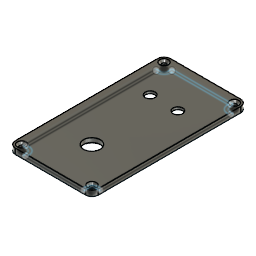
assembly (Autodesk Fusion 360 archive; units mm, degrees)
design "Couvercle"
part number: 2025-12-11-08-38-01-153
Autodesk Fusion 360 part; units mm, degrees
sketch "Esquisse1" plane through (0, 0, 0) normal (0, 0, 1) x (1, 0, 0)
  line L0 (0, 0) -> (60, 0)
  line L1 (60, 0) -> (60, -112)
  line L2 (60, -112) -> (0, -112)
  line L3 (0, -112) -> (0, 0)
  dimension "d1" = 60
  dimension "d2" = 112
  constraint horizontal L0
  constraint vertical L1
  constraint horizontal L2
  constraint vertical L3
  constraint coincident L0.start L3.end
  measures "d1" distance of L0.start L0.end
  measures "d2" distance of L0.start L2.end
extrude "Extrusion1" add sketch "Esquisse1" along normal blind 4
sketch "Esquisse2" plane through (0, 0, 4) normal (0, 0, 1) x (-1, 0, 0)
  line L0 (0, 112) -> (-60, 112)
  line L1 (-60, 112) -> (-60, 0)
  line L2 (-60, 0) -> (0, 0)
  line L3 (0, 0) -> (0, 112)
  circle A0 centre (-4.6, 4.6) radius 1.6
  circle A1 centre (-4.6, 4.6) radius 1.6
  circle A2 centre (-55.4, 4.6) radius 1.6
  circle A3 centre (-4.6, 107.4) radius 1.6
  circle A4 centre (-55.4, 107.4) radius 1.6
  dimension "d5" = 3.2
  dimension "d6" = 4.6
  dimension "d7" = 4.6
  dimension "d8" = 3.2
  dimension "d9" = 3.2
  dimension "d10" = 4.6
  dimension "d11" = 4.6
  dimension "d12" = 3.2
  dimension "d13" = 4.6
  dimension "d14" = 4.6
  dimension "d15" = 3.2
  dimension "d16" = 4.6
  dimension "d17" = 4.6
  measures "d5" diameter of A0
  measures "d6" distance of L3 A0.centre
  measures "d7" distance of L2 A0.centre
  measures "d8" diameter of A1
  measures "d9" diameter of A2
  measures "d10" distance of L1 A2.centre
  measures "d11" distance of L2 A2.centre
  measures "d12" diameter of A3
  measures "d13" distance of L0 A3.centre
  measures "d14" distance of L3 A3.centre
  measures "d15" diameter of A4
  measures "d16" distance of L1 A4.centre
  measures "d17" distance of L0 A4.centre
hole "Perçage1" at (4.6, -4.6, 4) at (55.4, -4.6, 4) at (55.4, -107.4, 4) at (4.6, -107.4, 4) direction (0, 0, -1) diameter 3.2 depth 25 tip angle 118 countersink diameter 6.3 countersink angle 90
fillet "Congé1" radius 4.6 4 edges at (0, 0, 2) (60, 0, 2) (60, -112, 2) (0, -112, 2)
sketch "Esquisse3" plane through (0, 0, 0) normal (0, 0, -1) x (1, 0, 0)
  circle A0 centre (55.4, 107.4) radius 1.6
  circle A1 centre (4.6, 4.6) radius 1.6
  circle A2 centre (55.4, 4.6) radius 1.6
  circle A3 centre (4.6, 107.4) radius 1.6
  arc A4 (4.6, 112) -> (0, 107.4) centre (4.6, 107.4) ccw
  line L0 (0, 107.4) -> (0, 4.6)
  arc A5 (0, 4.6) -> (4.6, 0) centre (4.6, 4.6) ccw
  line L1 (4.6, 0) -> (55.4, 0)
  arc A6 (55.4, 0) -> (60, 4.6) centre (55.4, 4.6) ccw
  line L2 (60, 4.6) -> (60, 107.4)
  arc A7 (60, 107.4) -> (55.4, 112) centre (55.4, 107.4) ccw
  line L3 (55.4, 112) -> (4.6, 112)
  line L4 (8.9, 110) -> (51.6, 110)
  line L5 (2, 8.7) -> (2, 103.1)
  line L6 (52.1, 107.4) -> (52.1, 109.5)
  arc A8 (52.1, 107.4) -> (55.4467, 104.1003) centre (55.4, 107.4) ccw
  line L7 (55.3533, 104.1003) -> (57.5, 104.1003)
  arc A9 (52.1, 109.5) -> (51.6, 110) centre (51.6, 109.5) ccw
  arc A10 (58, 103.6003) -> (57.5, 104.1003) centre (57.5, 103.6003) ccw
  line L8 (7.9, 109) -> (7.9, 107.4)
  line L9 (3, 104.1) -> (4.6, 104.1)
  arc A11 (4.6, 104.1) -> (7.9, 107.4) centre (4.6, 107.4) ccw
  line L10 (3, 7.7) -> (4.6, 7.7)
  line L11 (7.7, 3) -> (7.7, 4.6)
  arc A12 (7.7, 4.6) -> (4.6, 7.7) centre (4.6, 4.6) ccw
  line L12 (57, 7.7) -> (55.4, 7.7)
  line L13 (52.3, 3) -> (52.3, 4.6)
  arc A13 (55.4, 7.7) -> (52.3, 4.6) centre (55.4, 4.6) ccw
  line L14 (58, 103.6003) -> (58, 8.7)
  line L15 (51.3, 2) -> (8.7, 2)
  arc A14 (8.9, 110) -> (7.9, 109) centre (8.9, 109) ccw
  arc A15 (3, 104.1) -> (2, 103.1) centre (3, 103.1) ccw
  arc A16 (2, 8.7) -> (3, 7.7) centre (3, 8.7) ccw
  arc A17 (7.7, 3) -> (8.7, 2) centre (8.7, 3) ccw
  arc A18 (51.3, 2) -> (52.3, 3) centre (51.3, 3) ccw
  arc A19 (57, 7.7) -> (58, 8.7) centre (57, 8.7) ccw
  line L16 (55.4592, 102.1003) -> (56, 102.1003)
  line L17 (56, 102.1003) -> (56, 9.7)
  line L18 (56, 9.7) -> (55.4, 9.7)
  arc A20 (55.4, 9.7) -> (50.3, 4.6) centre (55.4, 4.6) ccw
  line L19 (50.3, 4) -> (50.3, 4.6)
  line L20 (50.3, 4) -> (9.7, 4)
  line L21 (9.7, 4) -> (9.7, 4.6)
  arc A21 (9.7, 4.6) -> (4.6, 9.7) centre (4.6, 4.6) ccw
  line L22 (4, 9.7) -> (4.6, 9.7)
  line L23 (4, 9.7) -> (4, 102.1)
  line L24 (4, 102.1) -> (4.6, 102.1)
  arc A22 (4.6, 102.1) -> (9.9, 107.4) centre (4.6, 107.4) ccw
  line L25 (9.9, 108) -> (9.9, 107.4)
  line L26 (9.9, 108) -> (50.1, 108)
  line L27 (50.1, 107.4) -> (50.1, 108)
  arc A23 (50.1, 107.4) -> (55.4592, 102.1003) centre (55.4, 107.4) ccw
  dimension "d25" = 2
  dimension "d27" = 2
  dimension "d28" = 2
  dimension "d30" = 0.5
  dimension "d31" = 0.5
  dimension "d36" = 1
  dimension "d37" = 2
  constraint horizontal L4
  constraint vertical L14
  constraint vertical L5
  constraint concentric A0 A8
  constraint perpendicular L4 L6
  constraint coincident A8 L7.start
  constraint horizontal L7
  constraint coincident L7 A8.end
  constraint tangent L4 A9
  constraint tangent L6 A9
  constraint tangent L7 A10
  constraint tangent A10 L14
  constraint concentric A3 A11
  constraint perpendicular L4 L8
  constraint tangent L8 A11
  constraint perpendicular L5 L9
  constraint tangent L9 A11
  constraint perpendicular L5 L10
  constraint concentric A1 A12
  constraint tangent L10 A12
  constraint tangent L11 A12
  constraint concentric A2 A13
  constraint perpendicular L12 L14
  constraint tangent L13 A13
  constraint tangent L12 A13
  constraint tangent L8 A14
  constraint tangent L4 A14
  constraint tangent L9 A15
  constraint tangent L5 A15
  constraint equal A14 A15
  constraint tangent L10 A16
  constraint tangent L5 A16
  constraint equal A14 A16
  constraint tangent L11 A17
  constraint tangent L15 A17
  constraint equal A14 A17
  constraint tangent L13 A18
  constraint tangent L15 A18
  constraint equal A14 A18
  constraint tangent L12 A19
  constraint tangent L14 A19
  constraint equal A14 A19
  measures "d25" distance of L3 L4
  measures "d27" distance of L2 L14
  measures "d28" distance of L0 L5
  measures "d30" radius of A9
  measures "d31" radius of A10
  measures "d36" radius of A14
sketch "Esquisse5" plane through (0, 0, 0) normal (0, 0, -1) x (1, 0, 0)
  circle A0 centre (30, 82.0769) radius 6
  dimension "d42" = 12
  measures "d42" diameter of A0
extrude "Extrusion4" cut sketch "Esquisse5" against normal blind 9
chamfer "Chanfrein1" distance 1 angle 45 1 edges at (24.406, -84.2466, 0)
extrude "Extrusion2" add sketch "Esquisse3" along normal blind 1.5 contours L4 L5 L6 A8 L7 A9 A10 L8 L9 A11 L10 L11 A12 L12 L13 A13 L14 L15 A14 A15 A16 A17 A18 A19
extrude "Extrusion3" cut 1 faces at (29.8256, -30.6684, 0) along direction (0, 0, 1) blind 2.2
sketch "Esquisse6" plane through (0, 0, 4) normal (0, 0, 1) x (-1, 0, 0)
  circle A0 centre (-30, 82.0769) radius 6
  arc A1 (0, 107.4) -> (-4.6, 112) centre (-4.6, 107.4) ccw
  line L0 (-4.6, 112) -> (-55.4, 112)
  arc A2 (-55.4, 112) -> (-60, 107.4) centre (-55.4, 107.4) ccw
  line L1 (-60, 107.4) -> (-60, 4.6)
  arc A3 (-60, 4.6) -> (-55.4, 0) centre (-55.4, 4.6) ccw
  line L2 (-55.4, 0) -> (-4.6, 0)
  arc A4 (-4.6, 0) -> (0, 4.6) centre (-4.6, 4.6) ccw
  line L3 (0, 4.6) -> (0, 107.4)
  circle A5 centre (-55.4, 107.4) radius 3.15
  circle A6 centre (-4.6, 4.6) radius 3.15
  circle A7 centre (-55.4, 4.6) radius 3.15
  circle A8 centre (-4.6, 107.4) radius 3.15
  circle A9 centre (-20, 30) radius 3.5
  circle A10 centre (-40, 30) radius 3.5
  dimension "d52" = 7
  dimension "d53" = 30
  dimension "d54" = 7
  dimension "d55" = 30
  dimension "d56" = 20
  dimension "d57" = 20
  measures "d52" diameter of A9
  measures "d53" distance of L2 A9.centre
  measures "d54" diameter of A10
  measures "d55" distance of L2 A10.centre
  measures "d56" distance of L1 A10.centre
  measures "d57" distance of L3 A9.centre
extrude "Extrusion5" cut sketch "Esquisse6" against normal blind 20 contours A9 | A10
equation "d6 = 3 mm + ( 3.2 / 2 ) * 1 mm"

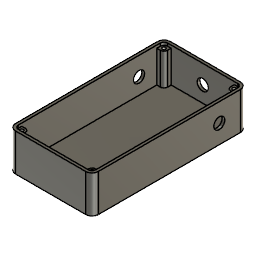
design "Boitier"
part number: 2025-12-11-09-13-35-348
Autodesk Fusion 360 part; units mm, degrees
sketch "Esquisse1" plane through (0, 0, 0) normal (0, 0, 1) x (1, 0, 0)
  line L0 (4.6, 0) -> (55.4, 0)
  line L1 (60, -4.6) -> (60, -107.4)
  line L2 (55.4, -112) -> (4.6, -112)
  line L3 (0, -107.4) -> (0, -4.6)
  arc A0 (1, 0) -> (0, -1) centre (1, -1) ccw
  arc A1 (60, -1) -> (59, 0) centre (59, -1) ccw
  arc A2 (59, -112) -> (60, -111) centre (59, -111) ccw
  arc A3 (0, -111) -> (1, -112) centre (1, -111) ccw
  arc A4 (4.6, 0) -> (0, -4.6) centre (4.6, -4.6) ccw
  arc A5 (55.4, -112) -> (60, -107.4) centre (55.4, -107.4) ccw
  arc A6 (60, -4.6) -> (55.4, 0) centre (55.4, -4.6) ccw
  arc A7 (0, -107.4) -> (4.6, -112) centre (4.6, -107.4) ccw
  point P0 (60, 0)
  point P1 (0, -112)
  dimension "d1" = 60
  dimension "d2" = 112
  dimension "d3" = 1
  dimension "d4" = 4.6
  constraint horizontal L0
  constraint vertical L1
  constraint horizontal L2
  constraint vertical L3
  constraint coincident origin L0
  constraint coincident origin L3
  constraint tangent L0 A0
  constraint tangent L3 A0
  constraint coincident P0 L0
  constraint coincident P0 L1
  constraint tangent L0 A1
  constraint tangent L1 A1
  constraint equal A0 A1
  constraint tangent L1 A2
  constraint tangent L2 A2
  constraint equal A0 A2
  constraint coincident P1 L3
  constraint coincident P1 L2
  constraint tangent L3 A3
  constraint tangent L2 A3
  constraint equal A0 A3
  constraint coincident L0 A0.start
  constraint coincident L3 A0.end
  constraint tangent L0 A4
  constraint tangent L3 A4
  constraint coincident L2 A2.start
  constraint coincident L1 A2.end
  constraint tangent L2 A5
  constraint tangent L1 A5
  constraint equal A4 A5
  constraint coincident L0 A1.end
  constraint coincident L1 A1.start
  constraint tangent L0 A6
  constraint tangent L1 A6
  constraint equal A4 A6
  constraint coincident L3 A3.start
  constraint coincident L2 A3.end
  constraint tangent L3 A7
  constraint tangent L2 A7
  constraint equal A4 A7
  measures "d1" distance of origin P0
  measures "d2" distance of origin P1
  measures "d3" radius of A0
  measures "d4" radius of A4
extrude "Extrusion1" add sketch "Esquisse1" along normal blind 2
shell "Coque1" thickness 25 removed faces 1 at (40, -38.8667, 2)
sketch "Esquisse2" plane through (0, 0, 2) normal (0, 0, 1) x (-1, 0, 0)
  arc A0 (-4.6, 0) -> (0, 4.6) centre (-4.6, 4.6) ccw
  line L0 (0, 4.6) -> (0, 107.4)
  arc A1 (0, 107.4) -> (-4.6, 112) centre (-4.6, 107.4) ccw
  line L1 (-4.6, 112) -> (-55.4, 112)
  arc A2 (-55.4, 112) -> (-60, 107.4) centre (-55.4, 107.4) ccw
  line L2 (-60, 107.4) -> (-60, 4.6)
  arc A3 (-60, 4.6) -> (-55.4, 0) centre (-55.4, 4.6) ccw
  line L3 (-55.4, 0) -> (-4.6, 0)
  line L4 (-4.6, 110) -> (-55.4, 110)
  arc A4 (-55.4, 110) -> (-58, 107.4) centre (-55.4, 107.4) ccw
  line L5 (-58, 107.4) -> (-58, 4.6)
  arc A5 (-58, 4.6) -> (-55.4, 2) centre (-55.4, 4.6) ccw
  line L6 (-55.4, 2) -> (-4.6, 2)
  arc A6 (-4.6, 2) -> (-2, 4.6) centre (-4.6, 4.6) ccw
  line L7 (-2, 4.6) -> (-2, 107.4)
  arc A7 (-2, 107.4) -> (-4.6, 110) centre (-4.6, 107.4) ccw
  dimension "d8" = -2
extrude "Extrusion2" add sketch "Esquisse2" along normal blind 25
sketch "Esquisse3" plane through (0, 0, 2) normal (0, 0, 1) x (-1, 0, 0)
  line L0 (-4.6, 110) -> (-55.4, 110)
  arc A0 (-55.4, 110) -> (-58, 107.4) centre (-55.4, 107.4) ccw
  line L1 (-58, 107.4) -> (-58, 4.6)
  arc A1 (-58, 4.6) -> (-55.4, 2) centre (-55.4, 4.6) ccw
  line L2 (-55.4, 2) -> (-4.6, 2)
  arc A2 (-4.6, 2) -> (-2, 4.6) centre (-4.6, 4.6) ccw
  line L3 (-2, 4.6) -> (-2, 107.4)
  arc A3 (-2, 107.4) -> (-4.6, 110) centre (-4.6, 107.4) ccw
  line L4 (-7.2, 2) -> (-7.2, 4.6)
  line L5 (-4.6, 7.2) -> (-2, 7.2)
  arc A4 (-4.6, 2) -> (-2, 4.6) centre (-4.6, 4.6) ccw
  arc A5 (-4.6, 7.2) -> (-7.2, 4.6) centre (-4.6, 4.6) ccw
  line L6 (-2, 104.8) -> (-4.6, 104.8)
  line L7 (-7.2, 107.4) -> (-7.2, 110)
  arc A6 (-7.2, 107.4) -> (-4.6, 104.8) centre (-4.6, 107.4) ccw
  arc A7 (-2, 107.4) -> (-4.6, 110) centre (-4.6, 107.4) ccw
  line L8 (-58, 104.8) -> (-55.4, 104.8)
  line L9 (-52.8, 107.4) -> (-52.8, 110)
  arc A8 (-55.4, 110) -> (-58, 107.4) centre (-55.4, 107.4) ccw
  arc A9 (-55.4, 104.8) -> (-52.8, 107.4) centre (-55.4, 107.4) ccw
  line L10 (-52.8, 2) -> (-52.8, 4.6)
  line L11 (-55.4, 7.2) -> (-58, 7.2)
  arc A10 (-52.8, 4.6) -> (-55.4, 7.2) centre (-55.4, 4.6) ccw
  arc A11 (-58, 4.6) -> (-55.4, 2) centre (-55.4, 4.6) ccw
  dimension "d11" = 2.6
  dimension "d12" = 2.6
  dimension "d13" = 5.2
  constraint coincident L2 L4.start
  constraint perpendicular L2 L4
  constraint coincident L3 L5.end
  constraint perpendicular L3 L5
  constraint tangent L4 A4
  constraint tangent L5 A4
  constraint coincident L5.start A4
  constraint concentric A4 A5
  constraint concentric A1 A10
  constraint concentric A0 A8
  constraint concentric A3 A6
  constraint coincident L3 L6.start
  constraint perpendicular L3 L6
  constraint coincident L0 L7.end
  constraint perpendicular L0 L7
  constraint tangent L6 A6
  constraint tangent L7 A6
  constraint concentric A6 A7
  constraint coincident L1 L8.start
  constraint perpendicular L1 L8
  constraint coincident L0 L9.end
  constraint perpendicular L0 L9
  constraint tangent L8 A8
  constraint tangent L9 A8
  constraint coincident L8.end A8
  constraint concentric A8 A9
  constraint coincident L2 L10.start
  constraint perpendicular L2 L10
  constraint coincident L1 L11.end
  constraint perpendicular L1 L11
  constraint tangent L10 A10
  constraint tangent L11 A10
  constraint concentric A10 A11
  measures "d11" distance of L2 A2.centre
  measures "d12" distance of L3 A2.centre
  measures "d13" diameter of A4
extrude "Extrusion3" add sketch "Esquisse3" along normal blind 23 contours L0 L3 A3 L6 L7 A6 A7 | L0 A0 L1 L8 L9 A8 A9 | L2 A2 L3 L4 L5 A4 A5 | L1 A1 L2 L10 L11 A10 A11
sketch "Esquisse4" plane through (0, 0, 25) normal (0, 0, 1) x (-1, 0, 0)
  arc A0 (-58, 4.6) -> (-55.4, 2) centre (-55.4, 4.6) ccw
  line L0 (-55.4, 2) -> (-52.8, 2)
  line L1 (-52.8, 2) -> (-52.8, 4.6)
  arc A1 (-52.8, 4.6) -> (-55.4, 7.2) centre (-55.4, 4.6) ccw
  line L2 (-55.4, 7.2) -> (-58, 7.2)
  line L3 (-58, 7.2) -> (-58, 4.6)
hole "Perçage1" at (55.4, -4.6, 25) direction (0, 0, -1) diameter 2.529 depth 10 tip angle 118
thread "Filetage1" "ISO Metric profile 3.0 M3x0.5 M3x0.5 6H" thread offset 0 thread depth 7.4
sketch "Esquisse5" plane through (0, 0, 25) normal (0, 0, 1) x (-1, 0, 0)
  line L0 (-7.2, 2) -> (-4.6, 2)
  arc A0 (-4.6, 2) -> (-2, 4.6) centre (-4.6, 4.6) ccw
  line L1 (-2, 4.6) -> (-2, 7.2)
  line L2 (-2, 7.2) -> (-4.6, 7.2)
  arc A1 (-4.6, 7.2) -> (-7.2, 4.6) centre (-4.6, 4.6) ccw
  line L3 (-7.2, 4.6) -> (-7.2, 2)
hole "Perçage2" at (4.6, -4.6, 25) direction (0, 0, -1) diameter 2.529 depth 10 tip angle 118
thread "Filetage2" "ISO Metric profile 3.0 M3x0.5 M3x0.5 6H" thread offset 0 thread depth 7.4
sketch "Esquisse6" plane through (0, 0, 25) normal (0, 0, 1) x (-1, 0, 0)
  line L0 (-2, 104.8) -> (-2, 107.4)
  arc A0 (-2, 107.4) -> (-4.6, 110) centre (-4.6, 107.4) ccw
  line L1 (-4.6, 110) -> (-7.2, 110)
  line L2 (-7.2, 110) -> (-7.2, 107.4)
  arc A1 (-7.2, 107.4) -> (-4.6, 104.8) centre (-4.6, 107.4) ccw
  line L3 (-4.6, 104.8) -> (-2, 104.8)
hole "Perçage3" at (4.6, -107.4, 25) direction (0, 0, -1) diameter 2.529 depth 10 tip angle 118
thread "Filetage3" "ISO Metric profile 3.0 M3x0.5 M3x0.5 6H" thread offset 0 thread depth 7.4
sketch "Esquisse7" plane through (0, 0, 25) normal (0, 0, 1) x (-1, 0, 0)
  arc A0 (-55.4, 104.8) -> (-52.8, 107.4) centre (-55.4, 107.4) ccw
  line L0 (-52.8, 107.4) -> (-52.8, 110)
  line L1 (-52.8, 110) -> (-55.4, 110)
  arc A1 (-55.4, 110) -> (-58, 107.4) centre (-55.4, 107.4) ccw
  line L2 (-58, 107.4) -> (-58, 104.8)
  line L3 (-58, 104.8) -> (-55.4, 104.8)
hole "Perçage4" at (55.4, -107.4, 25) direction (0, 0, -1) diameter 2.529 depth 10 tip angle 118
thread "Filetage4" "ISO Metric profile 3.0 M3x0.5 M3x0.5 6H" thread offset 0 thread depth 7.4
sketch "Esquisse10" plane through (0, 0, 0) normal (-1, 0, 0) x (0, -1, 0)
  line L0 (4.6, 0) -> (107.4, 0)
  line L1 (107.4, 0) -> (107.4, 27)
  line L2 (107.4, 27) -> (4.6, 27)
  line L3 (4.6, 27) -> (4.6, 0)
  circle A0 centre (20, 13.5) radius 4
  point P0 (0, 27)
  dimension "d58" = 8
  dimension "d59" = 13.5
  dimension "d60" = 20
  measures "d58" diameter of A0
  measures "d59" distance of L2 A0.centre
  measures "d60" horizontal distance of A0.centre P0
extrude "Extrusion4" cut sketch "Esquisse10" against normal blind 68 contours A0
sketch "Esquisse11" plane through (0, 0, 0) normal (0, 1, 0) x (-1, 0, 0)
  line L0 (-55.4, 0) -> (-4.6, 0)
  line L1 (-4.6, 0) -> (-4.6, 27)
  line L2 (-4.6, 27) -> (-55.4, 27)
  line L3 (-55.4, 27) -> (-55.4, 0)
  circle A0 centre (-30, 13.5) radius 4
  dimension "d63" = 8
  dimension "d64" = 25.4
  dimension "d65" = 13.5
  measures "d63" diameter of A0
  measures "d64" distance of L1 A0.centre
  measures "d65" distance of L2 A0.centre
extrude "Extrusion5" cut sketch "Esquisse11" against normal blind 24 contours A0
equation "d65 = ( 27 / 2 ) * 1 mm"
